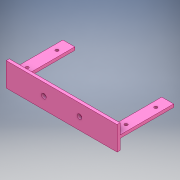
# Autodesk Inventor part: X-Axis Panel Mount
Saved by Autodesk Inventor 2018 (Build 220112000, 112)
## iProperties
Created: 2018-10-23
Part Number: X-Axis Panel Mount
Material: Steel
Document SubType Name: Modeling
Designer: P301319
Density: 7.85 g/cm^3
Appearance: Pink
Author: P301319
Autodesk Inventor part; units mm, degrees
ref_plane "YZ Plane" through (0, 0, 0) normal (1, 0, 0) x (0, 1, 0)
ref_plane "XZ Plane" through (0, 0, 0) normal (0, 1, 0) x (-1, 0, 0)
ref_plane "XY Plane" through (0, 0, 0) normal (0, 0, 1) x (1, 0, 0)
sketch "Sketch1" plane through (0, 0, 0) normal (0, 1, 0) x (-1, 0, 0)
  line L0 (0, 0) -> (-186, 0)
  line L1 (-186, 0) -> (-186, -40)
  line L2 (-186, -40) -> (0, -40)
  line L3 (0, -40) -> (0, 0)
  dimension "d0" = 186
  dimension "d1" = 40
  constraints: 8 end point, 2 parallel, 1 horizontal, 1 perpendicular
  measures "d0" distance of L2.end L1.end
  measures "d1" distance of L1.end L0.end
extrude "Extrusion1" add sketch "Sketch1" along normal blind 5
sketch "Sketch2" plane through (0, 5, 0) normal (0, 1, 0) x (1, 0, 0)
  line L0 (20, 17.5) -> (0, 17.5)
  line L1 (0, 17.5) -> (0, 22.5)
  line L2 (0, 22.5) -> (20, 22.5)
  line L3 (20, 22.5) -> (20, 17.5)
  line L4 (166, 22.5) -> (186, 22.5)
  line L5 (186, 22.5) -> (186, 17.5)
  line L6 (186, 17.5) -> (166, 17.5)
  line L7 (166, 17.5) -> (166, 22.5)
  line L8 (0, 40) -> (0, 0) projected
  line L9 (186, 0) -> (186, 40) projected
  point P0 (0, 20)
  point P1 (0, 20)
  point P2 (186, 20)
  point P3 (186, 20)
  point P4 (0, 20)
  point P5 (186, 20)
  dimension "d4" = 20
  dimension "d5" = 5
  dimension "d6" = 20
  dimension "d7" = 5
  constraints: 16 end point, 6 midpoint, 4 coincident, 4 parallel, 2 horizontal, 2 perpendicular
  measures "d4" distance of L1.end L2.end
  measures "d5" distance of L0.end L1.end
  measures "d6" distance of L5.end L6.end
  measures "d7" distance of L4.end L5.end
extrude "Extrusion2" add sketch "Sketch2" along normal blind 90
sketch "Sketch3" plane through (0, 5, 0) normal (0, 1, 0) x (1, 0, 0)
  circle A0 centre (63, 20) radius 4
  circle A1 centre (123, 20) radius 4
  line L0 (0, 22.5) -> (0, 17.5) projected
  line L1 (63, 20) -> (123, 20) construction
  line L2 (0, 0) -> (186, 0) projected
  point P0 (0, 20)
  point P1 (93, 20)
  point P2 (93, 0)
  dimension "d10" = 8
  dimension "d11" = 8
  dimension "d12" = 60
  constraints: 3 midpoint, 2 centre point, 2 end point, 2 horizontal alignment, 1 horizontal, 1 vertical alignment
  measures "d10" diameter of A0
  measures "d11" diameter of A1
  measures "d12" distance of L1.end L1.start
extrude "Extrusion3" cut sketch "Sketch3" against normal blind 90
sketch "Sketch4" plane through (166, 5, -17.5) normal (0, 0, 1) x (1, 0, 0)
  circle A0 centre (10, 20) radius 2.5
  circle A1 centre (10, 70) radius 2.5
  circle A2 centre (-156, 70) radius 2.5
  circle A3 centre (-156, 20) radius 2.5
  line L0 (0, 90) -> (20, 90) projected
  line L1 (-166, 90) -> (-146, 90) projected
  point P0 (-166, -5)
  point P1 (10, 90)
  point P2 (-156, 90)
  dimension "d17" = 5
  dimension "d18" = 5
  dimension "d19" = 5
  dimension "d20" = 5
  dimension "d21" = 50
  dimension "d22" = 50
  dimension "d23" = 20
  dimension "d24" = 20
  constraints: 4 centre point, 4 vertical alignment, 2 midpoint
  measures "d17" diameter of A0
  measures "d18" diameter of A1
  measures "d19" diameter of A2
  measures "d20" diameter of A3
  measures "d21" distance of A3.centre A2.centre
  measures "d22" distance of A0.centre A1.centre
  measures "d23" distance of point (-156, 90) A2.centre
  measures "d24" distance of point (10, 90) A1.centre
extrude "Extrusion4" cut sketch "Sketch4" against normal blind 90
equation "\"d22\" = d21"
equation "\"d24\" = d23"
body "Solid1"
